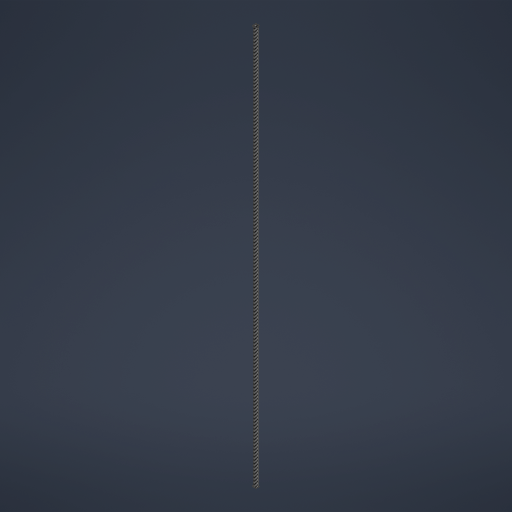
# Autodesk Inventor part: P_Wing_Carbonpipe_A
Saved by Autodesk Inventor 2026 (Build 300175000, 175)
## iProperties
Created: 2025-09-01
Part Number: P_Wing_Carbonpipe_A
Material: Generisch
Document SubType Name: Modeling
Designer: FAL
Density: 2.54648 g/cm^3
Appearance: Kohlenstofffaser
Mass: 20 g
Surface Area: 157.394 cm^2
Volume: 7.85398 cm^3
Author: FAL
Autodesk Inventor part; units mm, degrees
ref_plane "YZ Plane" through (0, 0, 0) normal (1, 0, 0) x (0, 1, 0)
ref_plane "XZ Plane" through (0, 0, 0) normal (0, 1, 0) x (-1, 0, 0)
ref_plane "XY Plane" through (0, 0, 0) normal (0, 0, 1) x (1, 0, 0)
sketch "Skizze1" plane through (0, 0, 0) normal (0, 0, 1) x (1, 0, 0)
  circle A0 centre (0, 0) radius 3
  circle A1 centre (0, 0) radius 2
  dimension "d0" = 1
  dimension "d1" = 6
  constraints: 2 centre point, 2 coincident
  measures "d0" radial gap between concentric circles of A0 A1
  measures "d1" diameter of A0
extrude "Extrusion1" add sketch "Skizze1" along normal mid plane 500
